Autodesk Inventor part; units mm, degrees
(part 2 of 2)
  line L927 (-1.7463, 34.8116) -> (-0.6604, 32.8106)
  line L928 (-0.6604, 32.8106) -> (0.7782, 31.0676)
  line L929 (0.7782, 31.0676) -> (2.5214, 29.6289)
  line L930 (2.5214, 29.6289) -> (4.5222, 28.5431)
  line L931 (4.5222, 28.5431) -> (6.7343, 27.8565)
  line L932 (6.7343, 27.8565) -> (8.5145, 27.617)
  line L933 (8.5145, 27.617) -> (9.1084, 27.617)
  line L934 (9.1084, 27.617) -> (9.701, 27.617)
  line L935 (9.701, 27.617) -> (11.4815, 27.8565)
  line L936 (11.4815, 27.8565) -> (13.6931, 28.5431)
  line L937 (13.6931, 28.5431) -> (15.6941, 29.6289)
  line L938 (15.6941, 29.6289) -> (17.4371, 31.0676)
  line L939 (17.4371, 31.0676) -> (18.8762, 32.8106)
  line L940 (18.8762, 32.8106) -> (19.9621, 34.8116)
  line L941 (19.9621, 34.8116) -> (20.6481, 37.0237)
  line L942 (20.6481, 37.0237) -> (20.8879, 38.8042)
  line L943 (20.8879, 38.8042) -> (20.8879, 39.396)
  line L944 (20.8879, 39.396) -> (20.8879, 39.9904)
  line L945 (20.8879, 39.9904) -> (20.6481, 41.7709)
  line L946 (20.6481, 41.7709) -> (19.9621, 43.9833)
  line L947 (19.9621, 43.9833) -> (18.8762, 45.9822)
  line L948 (18.8762, 45.9822) -> (17.4371, 47.7247)
  line L949 (17.4371, 47.7247) -> (15.6941, 49.1649)
  line L950 (15.6941, 49.1649) -> (13.6931, 50.2494)
  line L951 (13.6931, 50.2494) -> (11.4815, 50.9352)
  line L952 (11.4815, 50.9352) -> (9.701, 51.174)
  line L953 (9.701, 51.174) -> (9.1084, 51.174)
  line L954 (9.1084, 51.174) -> (8.5145, 51.174)
  line L955 (8.5145, 51.174) -> (6.7343, 50.9352)
  line L956 (6.7343, 50.9352) -> (4.5222, 50.2494)
  line L957 (4.5222, 50.2494) -> (2.5214, 49.1649)
  line L958 (2.5214, 49.1649) -> (0.7782, 47.7247)
  line L959 (0.7782, 47.7247) -> (-0.6604, 45.9822)
  line L960 (-0.6604, 45.9822) -> (-1.7463, 43.9833)
  line L961 (-1.7463, 43.9833) -> (-2.4326, 41.7709)
  line L962 (-2.4326, 41.7709) -> (-2.6711, 39.9904)
  line L963 (-2.6711, 39.9904) -> (-2.6711, 39.396)
  line L964 (9.336, 33.7808) -> (9.4957, 33.7808)
  line L965 (9.4957, 33.7808) -> (9.5755, 33.7808)
  line L966 (88.9063, 57.077) -> (88.6061, 57.0947)
  line L967 (88.6061, 57.0947) -> (87.3851, 57.1582)
  line L968 (87.3851, 57.1582) -> (86.5322, 57.2014)
  line L969 (86.5322, 57.2014) -> (86.4179, 57.2065)
  line L970 (86.4179, 57.2065) -> (86.4067, 57.2395)
  line L971 (86.4067, 57.2395) -> (86.2728, 57.6535)
  line L972 (86.2728, 57.6535) -> (85.9053, 58.8016)
  line L973 (85.9053, 58.8016) -> (85.3168, 60.6558)
  line L974 (85.3168, 60.6558) -> (84.7077, 62.5735)
  line L975 (84.7077, 62.5735) -> (84.505, 63.2136)
  line L976 (84.505, 63.2136) -> (82.857, 56.9855)
  line L977 (82.857, 56.9855) -> (80.5157, 56.7823)
  line L978 (80.5157, 56.7823) -> (77.8781, 68.9032)
  line L979 (77.8781, 68.9032) -> (78.2266, 68.9362)
  line L980 (78.2266, 68.9362) -> (79.646, 69.0632)
  line L981 (79.646, 69.0632) -> (80.63, 69.1521)
  line L982 (80.63, 69.1521) -> (80.7621, 69.1623)
  line L983 (80.7621, 69.1623) -> (80.8532, 68.5882)
  line L984 (80.8532, 68.5882) -> (81.7323, 62.8123)
  line L985 (81.7323, 62.8123) -> (81.8179, 62.2332)
  line L986 (81.8179, 62.2332) -> (83.0704, 68.258)
  line L987 (83.0704, 68.258) -> (85.7412, 67.9253)
  line L988 (85.7412, 67.9253) -> (87.2253, 63.2492)
  line L989 (87.2253, 63.2492) -> (88.3292, 69.7008)
  line L990 (88.3292, 69.7008) -> (91.4133, 69.4595)
  line L991 (91.4133, 69.4595) -> (88.9063, 57.077)
  line L992 (94.9561, 64.2067) -> (94.9713, 64.9078)
  line L993 (94.9713, 64.9078) -> (94.7257, 67.0109)
  line L994 (94.7257, 67.0109) -> (93.9447, 69.1547)
  line L995 (93.9447, 69.1547) -> (92.6863, 70.7193)
  line L996 (92.6863, 70.7193) -> (91.0287, 71.7886)
  line L997 (91.0287, 71.7886) -> (89.0458, 72.4414)
  line L998 (89.0458, 72.4414) -> (86.8133, 72.7564)
  line L999 (86.8133, 72.7564) -> (84.407, 72.8173)
  line L1000 (84.407, 72.8173) -> (82.5289, 72.7462)
  line L1001 (82.5289, 72.7462) -> (81.9048, 72.703)
  line L1002 (81.9048, 72.703) -> (81.0394, 72.6726)
  line L1003 (81.0394, 72.6726) -> (78.4639, 72.0249)
  line L1004 (78.4639, 72.0249) -> (76.0618, 70.3383)
  line L1005 (76.0618, 70.3383) -> (74.6673, 67.717)
  line L1006 (74.6673, 67.717) -> (74.2414, 65.111)
  line L1007 (74.2414, 65.111) -> (74.2579, 64.2448)
  line L1008 (74.2579, 64.2448) -> (74.2096, 63.3279)
  line L1009 (74.2096, 63.3279) -> (74.5154, 60.5466)
  line L1010 (74.5154, 60.5466) -> (75.7778, 57.5011)
  line L1011 (75.7778, 57.5011) -> (78.1619, 55.3726)
  line L1012 (78.1619, 55.3726) -> (80.8642, 54.4811)
  line L1013 (80.8642, 54.4811) -> (81.7806, 54.4201)
  line L1014 (81.7806, 54.4201) -> (82.4725, 54.3515)
  line L1015 (82.4725, 54.3515) -> (84.5601, 54.2576)
  line L1016 (84.5601, 54.2576) -> (87.1235, 54.3744)
  line L1017 (87.1235, 54.3744) -> (89.4166, 54.8291)
  line L1018 (89.4166, 54.8291) -> (91.3856, 55.6825)
  line L1019 (91.3856, 55.6825) -> (92.9772, 56.9906)
  line L1020 (92.9772, 56.9906) -> (94.1387, 58.8092)
  line L1021 (94.1387, 58.8092) -> (94.8154, 61.1943)
  line L1022 (94.8154, 61.1943) -> (94.9878, 63.4574)
  line L1023 (94.9878, 63.4574) -> (94.9561, 64.2067)
  line L1024 (104.8672, 60.5034) -> (104.6795, 60.5034)
  line L1025 (104.6795, 60.5034) -> (104.1186, 60.6101)
  line L1026 (104.1186, 60.6101) -> (103.5784, 60.9251)
  line L1027 (103.5784, 60.9251) -> (103.2451, 61.4508)
  line L1028 (103.2451, 61.4508) -> (103.1237, 62.002)
  line L1029 (103.1237, 62.002) -> (103.1194, 62.1874)
  line L1030 (103.1194, 62.1874) -> (103.1141, 62.3398)
  line L1031 (103.1141, 62.3398) -> (103.3579, 64.0721)
  line L1032 (103.3579, 64.0721) -> (103.413, 64.2652)
  line L1033 (103.413, 64.2652) -> (103.493, 64.5522)
  line L1034 (103.493, 64.5522) -> (104.0193, 65.586)
  line L1035 (104.0193, 65.586) -> (104.7183, 66.094)
  line L1036 (104.7183, 66.094) -> (104.8834, 66.1143)
  line L1037 (104.8834, 66.1143) -> (105.0363, 66.1346)
  line L1038 (105.0363, 66.1346) -> (105.5202, 66.0355)
  line L1039 (105.5202, 66.0355) -> (105.997, 65.6088)
  line L1040 (105.997, 65.6088) -> (106.3096, 64.8265)
  line L1041 (106.3096, 64.8265) -> (106.446, 63.9781)
  line L1042 (106.446, 63.9781) -> (106.4613, 63.6937)
  line L1043 (106.4613, 63.6937) -> (108.5339, 64.2652)
  line L1044 (108.5339, 64.2652) -> (108.5131, 64.4785)
  line L1045 (108.5131, 64.4785) -> (108.0874, 66.2921)
  line L1046 (108.0874, 66.2921) -> (108.0241, 66.4419)
  line L1047 (108.0241, 66.4419) -> (107.9152, 66.6909)
  line L1048 (107.9152, 66.6909) -> (107.4714, 67.3817)
  line L1049 (107.4714, 67.3817) -> (106.762, 68.0447)
  line L1050 (106.762, 68.0447) -> (105.8936, 68.4308)
  line L1051 (105.8936, 68.4308) -> (105.1219, 68.5425)
  line L1052 (105.1219, 68.5425) -> (104.8672, 68.5349)
  line L1053 (104.8672, 68.5349) -> (104.5804, 68.5273)
  line L1054 (104.5804, 68.5273) -> (103.2698, 68.0167)
  line L1055 (103.2698, 68.0167) -> (102.1179, 66.8788)
  line L1056 (102.1179, 66.8788) -> (101.9126, 66.5562)
  line L1057 (101.9126, 66.5562) -> (101.7153, 66.2489)
  line L1058 (101.7153, 66.2489) -> (101.0221, 64.5852)
  line L1059 (101.0221, 64.5852) -> (100.7092, 62.7589)
  line L1060 (100.7092, 62.7589) -> (100.7054, 62.3678)
  line L1061 (100.7054, 62.3678) -> (100.697, 61.9487)
  line L1062 (100.697, 61.9487) -> (101.018, 60.0945)
  line L1063 (101.018, 60.0945) -> (101.8187, 58.5679)
  line L1064 (101.8187, 58.5679) -> (102.0516, 58.3114)
  line L1065 (102.0516, 58.3114) -> (102.1674, 58.1844)
  line L1066 (102.1674, 58.1844) -> (102.9444, 57.7348)
  line L1067 (102.9444, 57.7348) -> (103.9106, 57.5418)
  line L1068 (103.9106, 57.5418) -> (104.2332, 57.5418)
  line L1069 (104.2332, 57.5418) -> (104.8065, 57.5418)
  line L1070 (104.8065, 57.5418) -> (106.5263, 57.8796)
  line L1071 (106.5263, 57.8796) -> (108.7681, 58.6594)
  line L1072 (108.7681, 58.6594) -> (109.2616, 58.8829)
  line L1073 (109.2616, 58.8829) -> (108.4112, 61.5651)
  line L1074 (108.4112, 61.5651) -> (108.0422, 61.3899)
  line L1075 (108.0422, 61.3899) -> (106.4173, 60.7701)
  line L1076 (106.4173, 60.7701) -> (105.254, 60.5034)
  line L1077 (105.254, 60.5034) -> (104.8672, 60.5034)
  line L1078 (122.0152, 66.1143) -> (122.0358, 66.1168)
  line L1079 (122.0358, 66.1168) -> (122.193, 66.1295)
  line L1080 (122.193, 66.1295) -> (122.2466, 66.1295)
  line L1081 (122.2466, 66.1295) -> (122.4671, 66.1295)
  line L1082 (122.4671, 66.1295) -> (123.1315, 65.7612)
  line L1083 (123.1315, 65.7612) -> (123.5738, 64.9027)
  line L1084 (123.5738, 64.9027) -> (123.6233, 64.6589)
  line L1085 (123.6233, 64.6589) -> (120.5766, 64.2982)
  line L1086 (120.5766, 64.2982) -> (120.6014, 64.57)
  line L1087 (120.6014, 64.57) -> (121.0119, 65.5631)
  line L1088 (121.0119, 65.5631) -> (121.8003, 66.0813)
  line L1089 (121.8003, 66.0813) -> (122.0152, 66.1143)
  line L1090 (124.289, 60.9454) -> (124.2215, 60.8438)
  line L1091 (124.2215, 60.8438) -> (123.4221, 60.1631)
  line L1092 (123.4221, 60.1631) -> (123.3297, 60.1275)
  line L1093 (123.3297, 60.1275) -> (123.2291, 60.0894)
  line L1094 (123.2291, 60.0894) -> (122.481, 59.8964)
  line L1095 (122.481, 59.8964) -> (122.2316, 59.8964)
  line L1096 (122.2316, 59.8964) -> (122.032, 59.8964)
  line L1097 (122.032, 59.8964) -> (121.4363, 60.0589)
  line L1098 (121.4363, 60.0589) -> (120.8466, 60.5466)
  line L1099 (120.8466, 60.5466) -> (120.461, 61.3619)
  line L1100 (120.461, 61.3619) -> (120.2984, 62.2128)
  line L1101 (120.2984, 62.2128) -> (120.2817, 62.4999)
  line L1102 (120.2817, 62.4999) -> (126.3312, 63.0536)
  line L1103 (126.3312, 63.0536) -> (126.3258, 63.3152)
  line L1104 (126.3258, 63.3152) -> (126.2032, 64.5115)
  line L1105 (126.2032, 64.5115) -> (125.9509, 65.5529)
  line L1106 (125.9509, 65.5529) -> (125.8821, 65.7384)
  line L1107 (125.8821, 65.7384) -> (125.7703, 66.0457)
  line L1108 (125.7703, 66.0457) -> (125.2908, 66.9118)
  line L1109 (125.2908, 66.9118) -> (124.4927, 67.75)
  line L1110 (124.4927, 67.75) -> (123.4884, 68.253)
  line L1111 (123.4884, 68.253) -> (122.5801, 68.4206)
  line L1112 (122.5801, 68.4206) -> (122.2784, 68.4206)
  line L1113 (122.2784, 68.4206) -> (122.1158, 68.4206)
  line L1114 (122.1158, 68.4206) -> (121.682, 68.3952)
  line L1115 (121.682, 68.3952) -> (121.6279, 68.3901)
  line L1116 (121.6279, 68.3901) -> (121.333, 68.3546)
  line L1117 (121.333, 68.3546) -> (120.0528, 67.7018)
  line L1118 (120.0528, 67.7018) -> (119.0249, 66.4191)
  line L1119 (119.0249, 66.4191) -> (118.8582, 66.066)
  line L1120 (118.8582, 66.066) -> (118.7904, 65.9212)
  line L1121 (118.7904, 65.9212) -> (118.2629, 64.2042)
  line L1122 (118.2629, 64.2042) -> (118.2243, 64.0035)
  line L1123 (118.2243, 64.0035) -> (118.205, 63.8969)
  line L1124 (118.205, 63.8969) -> (118.1153, 62.9342)
  line L1125 (118.1153, 62.9342) -> (118.1153, 62.6142)
  line L1126 (118.1153, 62.6142) -> (118.1153, 62.2255)
  line L1127 (118.1153, 62.2255) -> (118.2585, 61.0571)
  line L1128 (118.2585, 61.0571) -> (118.5923, 59.9472)
  line L1129 (118.5923, 59.9472) -> (118.6886, 59.749)
  line L1130 (118.6886, 59.749) -> (118.8222, 59.4747)
  line L1131 (118.8222, 59.4747) -> (119.747, 58.4206)
  line L1132 (119.747, 58.4206) -> (121.0134, 57.7983)
  line L1133 (121.0134, 57.7983) -> (121.3177, 57.7374)
  line L1134 (121.3177, 57.7374) -> (121.3924, 57.7221)
  line L1135 (121.3924, 57.7221) -> (122.0081, 57.6408)
  line L1136 (122.0081, 57.6408) -> (122.2149, 57.6408)
  line L1137 (122.2149, 57.6408) -> (122.525, 57.6408)
  line L1138 (122.525, 57.6408) -> (123.4595, 57.8186)
  line L1139 (123.4595, 57.8186) -> (124.5824, 58.352)
  line L1140 (124.5824, 58.352) -> (125.5801, 59.241)
  line L1141 (125.5801, 59.241) -> (126.2679, 60.158)
  line L1142 (126.2679, 60.158) -> (126.4554, 60.4856)
  line L1143 (126.4554, 60.4856) -> (124.5824, 61.5016)
  line L1144 (124.5824, 61.5016) -> (124.5621, 61.4508)
  line L1145 (124.5621, 61.4508) -> (124.3164, 60.986)
  line L1146 (124.3164, 60.986) -> (124.289, 60.9454)
  line L1147 (115.5677, 63.1196) -> (115.8346, 63.3406)
  line L1148 (115.8346, 63.3406) -> (116.8351, 64.7884)
  line L1149 (116.8351, 64.7884) -> (117.3822, 66.7188)
  line L1150 (117.3822, 66.7188) -> (117.4236, 67.1785)
  line L1151 (117.4236, 67.1785) -> (114.9322, 67.9126)
  line L1152 (114.9322, 67.9126) -> (114.939, 67.844)
  line L1153 (114.939, 67.844) -> (114.9792, 67.2827)
  line L1154 (114.9792, 67.2827) -> (114.9792, 67.0973)
  line L1155 (114.9792, 67.0973) -> (114.9792, 66.7925)
  line L1156 (114.9792, 66.7925) -> (114.8331, 65.8831)
  line L1157 (114.8331, 65.8831) -> (114.3975, 65.0018)
  line L1158 (114.3975, 65.0018) -> (113.6723, 64.4582)
  line L1159 (113.6723, 64.4582) -> (112.9134, 64.2601)
  line L1160 (112.9134, 64.2601) -> (112.6581, 64.2499)
  line L1161 (112.6581, 64.2499) -> (112.7823, 69.2766)
  line L1162 (112.7823, 69.2766) -> (109.9355, 69.081)
  line L1163 (109.9355, 69.081) -> (109.9355, 57.7374)
  line L1164 (109.9355, 57.7374) -> (112.5662, 57.7374)
  line L1165 (112.5662, 57.7374) -> (112.6581, 62.0249)
  line L1166 (112.6581, 62.0249) -> (112.7122, 62.0452)
  line L1167 (112.7122, 62.0452) -> (113.1351, 62.1392)
  line L1168 (113.1351, 62.1392) -> (113.2768, 62.1392)
  line L1169 (113.2768, 62.1392) -> (113.4633, 62.1392)
  line L1170 (113.4633, 62.1392) -> (114.0251, 61.8979)
  line L1171 (114.0251, 61.8979) -> (114.5519, 61.174)
  line L1172 (114.5519, 61.174) -> (114.8743, 59.9675)
  line L1173 (114.8743, 59.9675) -> (114.9982, 58.7026)
  line L1174 (114.9982, 58.7026) -> (115.0094, 58.2784)
  line L1175 (115.0094, 58.2784) -> (115.0119, 58.1387)
  line L1176 (115.0119, 58.1387) -> (115.0147, 57.331)
  line L1177 (115.0147, 57.331) -> (114.9487, 56.3429)
  line L1178 (114.9487, 56.3429) -> (114.9184, 56.1143)
  line L1179 (114.9184, 56.1143) -> (118.4765, 56.3759)
  line L1180 (118.4765, 56.3759) -> (118.4765, 56.7214)
  line L1181 (118.4765, 56.7214) -> (118.3909, 57.7628)
  line L1182 (118.3909, 57.7628) -> (118.1552, 58.8702)
  line L1183 (118.1552, 58.8702) -> (117.8095, 59.8532)
  line L1184 (117.8095, 59.8532) -> (117.495, 60.6101)
  line L1185 (117.495, 60.6101) -> (117.3932, 60.8641)
  line L1186 (117.3932, 60.8641) -> (117.2941, 61.0978)
  line L1187 (117.2941, 61.0978) -> (116.6411, 62.1316)
  line L1188 (116.6411, 62.1316) -> (115.7729, 62.9799)
  line L1189 (115.7729, 62.9799) -> (115.5677, 63.1196)
  line L1190 (96.5931, 67.1938) -> (96.2929, 57.8517)
  line L1191 (96.2929, 57.8517) -> (99.8606, 57.7221)
  line L1192 (99.8606, 57.7221) -> (99.363, 67.5875)
  line L1193 (99.363, 67.5875) -> (96.5931, 67.1938)
  line L1194 (131.9126, 64.6741) -> (131.7731, 64.603)
  line L1195 (131.7731, 64.603) -> (130.6474, 64.2321)
  line L1196 (130.6474, 64.2321) -> (130.2725, 64.2321)
  line L1197 (130.2725, 64.2321) -> (130.1069, 64.2321)
  line L1198 (130.1069, 64.2321) -> (129.6108, 64.3998)
  line L1199 (129.6108, 64.3998) -> (129.3202, 64.7909)
  line L1200 (129.3202, 64.7909) -> (129.2979, 64.9027)
  line L1201 (129.2979, 64.9027) -> (129.2842, 64.9637)
  line L1202 (129.2842, 64.9637) -> (129.2212, 65.5326)
  line L1203 (129.2212, 65.5326) -> (129.2212, 65.7206)
  line L1204 (129.2212, 65.7206) -> (129.2212, 66.0432)
  line L1205 (129.2212, 66.0432) -> (129.3284, 67.0033)
  line L1206 (129.3284, 67.0033) -> (129.5806, 68.1971)
  line L1207 (129.5806, 68.1971) -> (129.6535, 68.4536)
  line L1208 (129.6535, 68.4536) -> (127.147, 68.5857)
  line L1209 (127.147, 68.5857) -> (127.1031, 68.3774)
  line L1210 (127.1031, 68.3774) -> (126.8839, 66.6934)
  line L1211 (126.8839, 66.6934) -> (126.8839, 66.1295)
  line L1212 (126.8839, 66.1295) -> (126.8839, 65.7003)
  line L1213 (126.8839, 65.7003) -> (127.0627, 64.4074)
  line L1214 (127.0627, 64.4074) -> (127.6032, 63.1755)
  line L1215 (127.6032, 63.1755) -> (128.5019, 62.4338)
  line L1216 (128.5019, 62.4338) -> (129.447, 62.1874)
  line L1217 (129.447, 62.1874) -> (129.7627, 62.1874)
  line L1218 (129.7627, 62.1874) -> (130.0106, 62.1874)
  line L1219 (130.0106, 62.1874) -> (130.7589, 62.2992)
  line L1220 (130.7589, 62.2992) -> (131.6959, 62.5583)
  line L1221 (131.6959, 62.5583) -> (131.8973, 62.6294)
  line L1222 (131.8973, 62.6294) -> (131.8765, 62.2789)
  line L1223 (131.8765, 62.2789) -> (131.7277, 61.2349)
  line L1224 (131.7277, 61.2349) -> (131.4051, 60.2697)
  line L1225 (131.4051, 60.2697) -> (130.9296, 59.7363)
  line L1226 (130.9296, 59.7363) -> (130.4503, 59.6119)
  line L1227 (130.4503, 59.6119) -> (130.3027, 59.6347)
  line L1228 (130.3027, 59.6347) -> (130.143, 59.6601)
  line L1229 (130.143, 59.6601) -> (129.5834, 60.1021)
  line L1230 (129.5834, 60.1021) -> (129.3436, 60.9301)
  line L1231 (129.3436, 60.9301) -> (129.3436, 61.207)
  line L1232 (129.3436, 61.207) -> (129.3436, 61.3061)
  line L1233 (129.3436, 61.3061) -> (129.3573, 61.5651)
  line L1234 (129.3573, 61.5651) -> (129.3601, 61.6007)
  line L1235 (129.3601, 61.6007) -> (126.9926, 61.2883)
  line L1236 (126.9926, 61.2883) -> (127.001, 60.8463)
  line L1237 (127.001, 60.8463) -> (127.2021, 59.5204)
  line L1238 (127.2021, 59.5204) -> (127.7546, 58.2047)
  line L1239 (127.7546, 58.2047) -> (128.6492, 57.3437)
  line L1240 (128.6492, 57.3437) -> (129.5697, 56.9779)
  line L1241 (129.5697, 56.9779) -> (129.8864, 56.9373)
  line L1242 (129.8864, 56.9373) -> (129.9238, 56.9322)
  line L1243 (129.9238, 56.9322) -> (130.242, 56.9042)
  line L1244 (130.242, 56.9042) -> (130.3497, 56.9042)
  line L1245 (130.3497, 56.9042) -> (130.7343, 56.9042)
  line L1246 (130.7343, 56.9042) -> (131.8887, 57.3132)
  line L1247 (131.8887, 57.3132) -> (132.9278, 58.2682)
  line L1248 (132.9278, 58.2682) -> (133.1041, 58.54)
  line L1249 (133.1041, 58.54) -> (133.2298, 58.7407)
  line L1250 (133.2298, 58.7407) -> (133.7216, 59.8151)
  line L1251 (133.7216, 59.8151) -> (134.0292, 61.0038)
  line L1252 (134.0292, 61.0038) -> (134.0634, 61.2553)
  line L1253 (134.0634, 61.2553) -> (134.1061, 61.6007)
  line L1254 (134.1061, 61.6007) -> (134.3141, 64.1153)
  line L1255 (134.3141, 64.1153) -> (134.5057, 67.6942)
  line L1256 (134.5057, 67.6942) -> (134.5432, 68.5679)
  line L1257 (134.5432, 68.5679) -> (131.8821, 68.3215)
  line L1258 (131.8821, 68.3215) -> (131.9126, 64.6741)
  line L1259 (113.351, 12.7296) -> (96.6919, 29.3884)
  line L1260 (112.6439, 12.0224) -> (95.9848, 28.6813)
  line L1261 (95.9848, 12.7293) -> (112.6436, 29.3884)
  line L1262 (96.6919, 12.0222) -> (113.3507, 28.6813)
  line L1263 (112.6439, 12.0224) -> (113.351, 12.7296)
  line L1264 (96.6919, 12.0222) -> (95.9848, 12.7293)
  line L1265 (96.6919, 29.3884) -> (95.9848, 28.6813)
  line L1266 (113.3507, 28.6813) -> (112.6436, 29.3884)
  point P0 (105.375, 20.7054)
  point P1 (104.6679, 19.9983)
  point P2 (103.9608, 20.7054)
  point P3 (104.6679, 21.4125)
  dimension "d76" = 0.5
  dimension "d77" = 0.5
  dimension "d78" = 0.5
  dimension "d79" = 0.5
  constraints: 2534 end point, 4 parallel, 3 perpendicular, 1 point on line
  measures "d76" distance between parallel lines of L707 L1259
  measures "d77" distance between parallel lines of L707 L1260
  measures "d78" distance between parallel lines of L702 L1261
  measures "d79" distance between parallel lines of L702 L1262
extrude "Extrusion25" add sketch "Sketch1" along normal blind 0.25 contours L621 L620 L619 L618 L617 L616 L615 L614 L613 L612 L611 L610 L609 L608 L607 L606 L605 L604 L603 L602 L601 L600 L599 L598 L597 L596 L595 L594 L593 L592 L591 L590 L589 L588 L587 L586 L585 L584 L583 L582 L581 L580 L579 L578 L577 L576 L575 L574 L573 L572 L571 L570 L569 L568 L567 L566 L565 L564 L563 L562 L561 L560 L559 L558 L557 L556 L555 L554 L553 L552 L551 L550 L549 L548 L547 L546 L545 L544 L543 L542 L541 L540 L539 L538 L537 L536 L535 L534 L533 L532 L531 L530 L529 L528 L527 L526 L525 L524 L523 L522 L521 L520 L519 L518 L517 L516 L515 L514 L513 L512 L511 L510 L509 L508 L507 L506 L505 L504 L503 L502 L501 L500 L499 L498 L497 L496 L495 L494 L493 L492 L491 L490 L489 L488 L487 L486 L485 L484 L483 L482 L481 L480 L479 L478 L477 L476 L475 L474 L473 L472 L471 L470 L469 L468 L467 L466 L465 L464 L463 L462 L461 L460 L459 L458 L457 L456 L455 L454
extrude "Extrusion26" add sketch "Sketch1" along normal blind 0.5 contours L919 L918 L917 L916 L915 L51 L50 | L50 L51 L915 L914 L913 L912 L911 L910 L909 L908 L907 L906 L905 L904 L903 L902 L901 L900 L899 L898 L897 L896 L895 L894 L893 L892 L891 L890 L889 L888 L887 L886 L885 L884 L923 L922 L921 L920 L919 | L790 L789 L788 L787 L786 L785 L784 L783 L68 L67 L66 L65 L64 L63 L62 L61 L60 L59 L58 L57 | L57 L58 L59 L60 L61 L62 L63 L64 L65 L66 L67 L68 L783 L782 L781 L780 L779 L778 L777 L776 L775 L774 L773 L772 L771 L770 L769 L768 L767 L766 L765 L764 L763 L762 L761 L760 L759 L758 L757 L796 L795 L794 L793 L792 L791 L790 | L832 L831 L830 L829 L828 L75 L74 | L74 L75 L828 L827 L826 L825 L824 L823 L822 L821 L820 L819 L818 L817 L816 L815 L814 L813 L812 L811 L810 L809 L808 L807 L806 L805 L804 L843 L842 L841 L840 L839 L838 L837 L836 L835 L834 L833 L832 | L104 L105 L106 L107 L108 L109 L110 L111 L112 L113 L114 L115 L116 L117 L118 L119 L120 L121 L122 L123 L124 L125 L126 L127 L128 L129 L130 L131 L132 L133 L134 L135 L136 L137 L138 L139 L140 L141 L142 L143 L144 L145 L146 L147 L148 L149 L150 L151 L152 L153 L154 L155 L156 L157 L158 L159 L160 L161 L162 L163 L164 L165 L166 L167 L168 L169 L170 L171 L172 L173 L174 L175 L176 L177 L178 L179 L180 L181 L182 L183 L184 L185 L186 L187 L188 L189 L190 L191 L192 L193 L194 L195 L196 L197 L198 L199 L200 L201 L202 L203 L204 L205 L206 L207 L208 L209 L210 L211 L212 L213 L214 L215 L216 L217 L218 L219 L220 L221 L222 L223 L224 L225 L226 L227 L228 L229 L230 L231 L232 L233 L234 L235 L236 L237 L238 L239 L240 L241 L242 L243 L244 L245 L246 L247 L248 L249 L250 L251 L252 L253 L254 L255 L256 L257 L258 L259 L260 L261 L262 L263 L264 L265 L266 L267 L268 L269 L270 L271 L272 L273 L274 L275 L276 L277 L278 L279 L280 L281 L282 L283 L284 L285 L286 L287 L288 L289 L290 L291 L292 L293 L294 L295 L296 L297 L298 L299 L300 L301 L302 L303 L304 L305 L306 L307 L308 L309 L310 L311 L312 L313 L314 L315 L316 L317 L318 L319 L320 L321 L322 L323 L324 L325 L326 L327 L328 L329 L330 L331 L332 L333 L334 L335 L336 L337 L338 L339 L340 L341 L342 L343 L344 L345 L346 L347 L348 L349 L350 L351 L352 L353 L354 L355 L356 L357 L358 L359 L360 L361 L362 L363 L364 L365 L366 L367 L368 L369 L370 L371 L372 L373 L374 L375 L376 L377 L378 L379 L380 L381 L382 L383 L384 L385 L386 L387 L388 L389 L390 L391 L392 L393 L394 L395 L396 L397 L398 L399 L400 L401 L402 L403 L404 L405 L406 L407 L408 L409 L410 L411 L412 L413 L414 L415 L416 L417 L418 L419 L420 L421 L422 L423 L424 L425 L426 L427 L428 L429 L430 L431 L432 L433 L434 L435 L436 L437 L438 L439 L440 L441 L442 L443 L444 L445 L446 L447 L448 L449 L450 L451 L452 L453 | L622 L623 L624 L625 L626 L627 L628 L629 L630 L631 L632 L633 L634 L635 L636 L637 L638 L639 L640 L641 L642 L643 L644 L645 L646 L647 L648 L649 L650 L651 L652 L653 L654 L655 L656 L657 L658 L659 L660 L661 | L701 L700 L699 L698 L697 L696 L695 L694 L693 L692 L691 L690 L689 L688 L687 L686 L685 L684 L683 L682 L681 L680 L679 L678 L677 L676 L675 L674 L673 L672 L671 L670 L669 L668 L667 L666 L665 L664 L663 L662 | L712 L713 L714 L715 L716 L717 L718 L719 L720 L721 L722 L723 L724 L725 L726 L727 L728 L729 L730 L731 L732 L733 L734 L735 L736 L737 L738 L739 L740 L741 L742 L743 L744 L745 L746 L747 L748 L749 L750 L751 | L883 L882 L881 L880 L879 L878 L877 L876 L875 L874 L873 L872 L871 L870 L869 L868 L867 L866 L865 L864 L863 L862 L861 L860 L859 L858 L857 L856 L855 L854 L853 L852 L851 L850 L849 L848 L847 L846 L845 L844 | L963 L962 L961 L960 L959 L958 L957 L956 L955 L954 L953 L952 L951 L950 L949 L948 L947 L946 L945 L944 L943 L942 L941 L940 L939 L938 L937 L936 L935 L934 L933 L932 L931 L930 L929 L928 L927 L926 L925 L924 | L966 L967 L968 L969 L970 L971 L972 L973 L974 L975 L976 L977 L978 L979 L980 L981 L982 L983 L984 L985 L986 L987 L988 L989 L990 L991 | L1078 L1079 L1080 L1081 L1082 L1083 L1084 L1085 L1086 L1087 L1088 L1089
body "Solid5"
